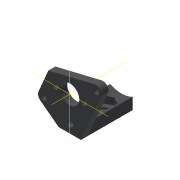
# Autodesk Inventor part: empty
Saved by Autodesk Inventor 2014 (Build 180170000, 170)
## iProperties
Created: 2015-04-13
Part Number: empty
Material: Generic
Document SubType Name: Modeling
Designer: Martin
Density: 1 g/cm^3
Appearance: Default
Author: Martin
Autodesk Inventor part; units mm, degrees
ref_plane "YZ Plane" through (0, 0, 0) normal (1, 0, 0) x (0, 1, 0)
ref_plane "XZ Plane" through (0, 0, 0) normal (0, 1, 0) x (-1, 0, 0)
sketch "sk_base" plane through (0, 0, 0) normal (0, 1, 0) x (-1, 0, 0)
  line L0 (16.4021, 0) -> (-16.8737, 0) projected
  line L1 (0, -22.2) -> (0, 14.2) projected
  circle A0 centre (0, 0) radius 8.8 construction
  circle A1 centre (0, -9) radius 1.2
  circle A2 centre (5.075, 0) radius 1
  circle A3 centre (-5.075, 0) radius 1
  circle A4 centre (0, 0) radius 3.4
  line L2 (9.4, -5.5883) -> (-9.4, 5.5883) construction
  circle A5 centre (9.4, -5.5883) radius 1 construction
  circle A6 centre (-9.4, 5.5883) radius 1 construction
  circle A7 centre (0, 0) radius 9 construction
  circle A8 centre (0, -9) radius 8 construction
  circle A9 centre (9.4, -5.5883) radius 2 construction
  circle A10 centre (-9.4, 5.5883) radius 2 construction
  line L3 (-8.6663, 7.4488) -> (8.9868, 0.4877)
  line L4 (8.9868, 0.4877) -> (11.2402, -4.8048)
  line L5 (4, -8.0623) -> (4, -12.2) construction
  line L6 (4, -12.2) -> (-4, -12.2)
  line L7 (-4, -12.2) -> (-4, -8.0623) construction
  line L8 (4, -9) -> (-4, -9) construction
  line L9 (4, -12.2) -> (10.6095, -7.1811)
  arc A11 (10.6095, -7.1811) -> (11.2402, -4.8048) centre (9.4, -5.5883) ccw
  line L10 (-11.2402, 4.8048) -> (-6.8151, -5.5883)
  line L11 (9.4, -5.5883) -> (-6.8151, -5.5883) construction
  arc A12 (-8.6663, 7.4488) -> (-11.2402, 4.8048) centre (-9.4, 5.5883) ccw
  line L12 (7.6889, 3.536) -> (-8.9324, 7.5328)
  line L13 (-4, -12.2) -> (-6.8151, -5.5883)
  line L14 (7.6889, 3.536) -> (8.9868, 0.4877)
  circle A13 centre (9.4, -5.5883) radius 1
  circle A14 centre (-9.4, 5.5883) radius 1
  dimension "d0" = 17.6
  dimension "d1" = 10.15
  dimension "d2" = 2
  dimension "d3" = 6.8
  dimension "servo_dowel_diameter" = 2.4
  dimension "servo_distance_gearcenters" = 9
  dimension "d7" = 18
  dimension "d8" = 16
  dimension "d10" = 4
  dimension "d11" = 3.2
  dimension "d12" = 8
  dimension "d13" = 8
  dimension "d16" = 9.4
  dimension "m2_screw_selfthreading_hole_diam" = 2
  constraints: 26 end point, 15 centre point, 13 point on circle, 9 coincident, 8 tangent, 5 equal radius, 5 parallel, 5 point on line, 2 perpendicular, 1 collinear, 1 midpoint, 2 other
  measures "d0" diameter of A0
  measures "d1" distance of A3.centre A2.centre
  measures "d2" diameter of A2
  measures "d3" diameter of A4
  measures "servo_dowel_diameter" diameter of A1
  measures "servo_distance_gearcenters" distance of A1.centre point (0, 0)
  measures "d7" diameter of A7
  measures "d8" diameter of A8
  measures "d10" diameter of A10
  measures "d11" distance between parallel lines of L6 L8
  measures "d12" distance between parallel lines of L7 L5
  measures "d13" angle of L3 L12
  measures "d16" distance from line of L1 L2.start
  measures "m2_screw_selfthreading_hole_diam" diameter of A14
extrude "ext_front" add sketch "sk_base" along normal blind 2.5 contours L4 A11 L9 L6 L1 A1 A4 L0 A2 | L0 A2 A4 L1 L3 L4 | L3 L1 L12 L14 | L3 A12 L12 L1 | L1 A4 L0 A3 L10 A12 L3 | L1 A1 L6 L13 L10 L0 A3 A4
sketch "Sketch2" plane through (0, 2.5, 0) normal (0, 1, 0) x (1, 0, 0)
  line L0 (-4, 8.0623) -> (-4, 12.2) construction
  line L1 (-4, 9) -> (4, 9) construction
  line L2 (4, 12.2) -> (4, 8.0623) construction
  circle A0 centre (0, 0) radius 9 construction
  line L3 (4, 12.2) -> (-4, 12.2)
  line L4 (-4, 12.2) -> (-4, 9)
  line L5 (-4, 9) -> (4, 9)
  line L6 (4, 9) -> (4, 12.2)
  arc A1 (4, 8.0623) -> (-4, 8.0623) centre (0, 0) ccw
  line L7 (4, 8.0623) -> (4, 9)
  line L8 (-4, 8.0623) -> (-4, 9)
  constraints: 12 end point, 3 point on circle, 2 parallel, 2 perpendicular, 1 centre point, 1 collinear, 1 concentric, 1 horizontal
extrude "ext_backsupport" add sketch "Sketch2" along normal blind 16
ref_plane "Work Plane1" through (0, 18.5, -9) normal (0, 0, 1) x (1, 0, 0)
sketch "sk_mounthole" plane through (0, 18.5, -9) normal (0, 0, 1) x (1, 0, 0)
  line L0 (-1.1973, -16) -> (1.1973, -16) projected
  line L1 (0, -22.2) -> (0, 3.7) projected
  circle A0 centre (0, -6) radius 1.5
  line L2 (0, -2.5359) -> (-3, -4.2679)
  line L3 (-3, -4.2679) -> (-3, -7.7321)
  line L4 (-3, -7.7321) -> (0, -9.4641)
  line L5 (0, -9.4641) -> (3, -7.7321)
  line L6 (3, -7.7321) -> (3, -4.2679)
  line L7 (3, -4.2679) -> (0, -2.5359)
  line L8 (-3, -6) -> (3, -6) construction
  point P0 (0, -18.5)
  dimension "m3_screw_max_diam" = 3
  dimension "d23" = 120
  dimension "d24" = 10
  constraints: 14 end point, 5 equal length, 3 midpoint, 3 parallel, 3 point on line, 1 centre point
  measures "m3_screw_max_diam" diameter of A0
  measures "d23" angle of L7 L2
  measures "d24" distance from line of L0 A0.centre
extrude "ext_mounthole" cut sketch "sk_mounthole" along normal through all both and the other way through all contours A0 L1 | L1 A0
extrude "ext_mountnut" cut sketch "sk_mounthole" along normal blind 10 and the other way blind 2.4
equation "\"d2\" = screw_m2_bore_selfthreading"
equation "\"servo_dowel_diameter\" = general_dowel_diameter"
equation "\"m2_screw_selfthreading_hole_diam\" = screw_m2_bore_selfthreading"
equation "\"screw_m2_bore_selfthreading\" = 2"
equation "\"general_dowel_diameter\" = 2.4"
body "Solid1"
